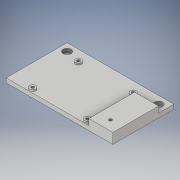
# Autodesk Inventor part: SF GPS
Saved by Autodesk Inventor 2019 (Build 230136000, 136)
## iProperties
Created: 2020-08-03
Part Number: SF GPS
Material: Generic
Document SubType Name: Modeling
Designer: james
Density: 1 g/cm^3
Appearance: Default
Author: james
Autodesk Inventor part; units mm, degrees
ref_plane "YZ Plane" through (0, 0, 0) normal (1, 0, 0) x (0, 1, 0)
ref_plane "XZ Plane" through (0, 0, 0) normal (0, 1, 0) x (-1, 0, 0)
ref_plane "XY Plane" through (0, 0, 0) normal (0, 0, 1) x (1, 0, 0)
sketch "Sketch1" plane through (0, 0, 0) normal (0, 1, 0) x (-1, 0, 0)
  line L0 (49.0764, 56.1521) -> (-39.8236, 56.1521)
  line L1 (-39.8236, 56.1521) -> (-39.8236, 5.3521)
  line L2 (-39.8236, 5.3521) -> (49.0764, 5.3521)
  line L3 (49.0764, 5.3521) -> (49.0764, 56.1521)
  point P0 (0, 0)
  dimension "d0" = 88.9
  dimension "d1" = 50.8
  constraints: 8 end point, 2 parallel, 1 horizontal, 1 perpendicular
  measures "d0" distance of L1.end L2.end
  measures "d1" distance between parallel lines of L0 L2
extrude "Extrusion1" add sketch "Sketch1" along normal blind 3.556
sketch "Sketch2" plane through (0, 3.556, 0) normal (0, 1, 0) x (1, 0, 0)
  line L0 (39.8236, -56.1521) -> (39.8236, -5.3521) projected
  line L1 (39.8236, -5.3521) -> (-49.0764, -5.3521) projected
  point P0 (0, 0)
  point P1 (-42.7264, -11.7021)
  point P2 (33.4736, -11.7021)
  dimension "d4" = 76.2
  dimension "d5" = 0
  dimension "d6" = 6.35
  dimension "d7" = 6.35
  measures "d4" distance of point (33.474, -11.702) point (-42.726, -11.702)
  measures "d5" vertical distance of point (-42.726, -11.702) point (33.474, -11.702)
  measures "d6" distance from line of point (33.474, -11.702) L0
  measures "d7" distance from line of L1 point (33.474, -11.702)
hole "Hole1" at (-42.7264, 3.556, 11.7021) at (33.4736, 3.556, 11.7021) direction (0, -1, 0) diameter 6.6548 end through all
sketch "Sketch3" plane through (0, 3.556, 0) normal (0, 1, 0) x (1, 0, 0)
  circle A0 centre (-30.0264, -53.1041) radius 2.54
  circle A1 centre (-30.0264, -15.0041) radius 2.54
  line L0 (-49.0764, -56.1521) -> (39.8236, -56.1521) projected
  line L1 (-49.0764, -5.3521) -> (-49.0764, -56.1521) projected
  circle A2 centre (15.6936, -53.1041) radius 2.54
  circle A3 centre (15.6936, -15.0041) radius 2.54
  point P0 (0, 0)
  dimension "d15" = 5.08
  dimension "d16" = 5.08
  dimension "d17" = 3.048
  dimension "d18" = 38.1
  dimension "d19" = 0
  dimension "d20" = 19.05
  dimension "d21" = 5.08
  dimension "d22" = 0
  dimension "d23" = 45.72
  dimension "d24" = 5.08
  dimension "d25" = 0
  dimension "d26" = 0
  constraints: 4 centre point
  measures "d15" diameter of A0
  measures "d16" diameter of A1
  measures "d17" distance from line of L0 A0.centre
  measures "d18" distance of A0.centre A1.centre
  measures "d19" horizontal distance of A0.centre A1.centre
  measures "d20" distance from line of L1 A0.centre
  measures "d21" diameter of A2
  measures "d22" vertical distance of A2.centre A0.centre
  measures "d23" distance of A2.centre A0.centre
  measures "d24" diameter of A3
  measures "d25" vertical distance of A3.centre A1.centre
  measures "d26" horizontal distance of A2.centre A3.centre
extrude "Extrusion2" add sketch "Sketch3" along normal blind 1.27
sketch "Sketch4" plane through (-30.0264, 4.826, 15.0041) normal (0, 1, 0) x (1, 0, 0)
  circle A0 centre (0, 0) radius 2.54 projected
  circle A1 centre (0, -38.1) radius 2.54 projected
  circle A2 centre (45.72, -38.1) radius 2.54 projected
  circle A3 centre (45.72, 0) radius 2.54 projected
  circle A4 centre (45.72, 0) radius 2.54 projected
  circle A5 centre (45.72, -38.1) radius 2.54 projected
  point P0 (30.0264, 15.0041)
  point P1 (45.72, 0)
  constraints: 4 coincident
hole "Hole2" at (-30.0264, 4.826, 53.1041) at (-30.0264, 4.826, 15.0041) at (15.6936, 4.826, 15.0041) at (15.6936, 4.826, 53.1041) direction (0, -1, 0) diameter 2.4638 end through all
sketch "Sketch5" plane through (0, 3.556, 0) normal (0, 1, 0) x (1, 0, 0)
  line L0 (19.8236, -18.0521) -> (39.8236, -18.0521)
  line L1 (39.8236, -18.0521) -> (39.8236, -56.1521)
  line L2 (39.8236, -56.1521) -> (19.8236, -56.1521)
  line L3 (19.8236, -56.1521) -> (19.8236, -18.0521)
  line L4 (39.8236, -56.1521) -> (39.8236, -5.3521) projected
  line L5 (-49.0764, -56.1521) -> (39.8236, -56.1521) projected
  line L6 (39.8236, -5.3521) -> (-49.0764, -5.3521) projected
  point P0 (0, 0)
  dimension "d36" = 0
  dimension "d37" = 20
  dimension "d38" = 0
  dimension "d40" = 12.7
  constraints: 8 end point, 2 parallel, 1 horizontal, 1 perpendicular
  measures "d36" distance between parallel lines of L4 L1
  measures "d37" distance of L1.end L2.end
  measures "d38" distance between parallel lines of L5 L2
  measures "d40" distance between parallel lines of L0 L6
extrude "Extrusion3" add sketch "Sketch5" along normal blind 5.08
sketch "Sketch6" plane through (0, 8.636, 0) normal (0, 1, 0) x (1, 0, 0)
  line L0 (19.8236, -56.1521) -> (39.8236, -56.1521) projected
  line L1 (39.8236, -56.1521) -> (39.8236, -18.0521) projected
  point P0 (0, 0)
  point P1 (29.8236, -48.1521)
  dimension "d43" = 8
  dimension "d44" = 10
  measures "d43" distance from line of L0 point (29.824, -48.152)
  measures "d44" distance from line of L1 point (29.824, -48.152)
hole "Hole3" at (29.8236, 8.636, 48.1521) direction (0, -1, 0) diameter 2.4638 end through all
body "Solid1"
